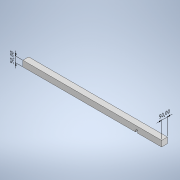
# Autodesk Inventor part: u_lange_Stange
Saved by Autodesk Inventor 2020.3 (Build 243373000, 373)
## iProperties
Created: 2020-09-30
Part Number: u_lange_Stange
Material: Generic
Document SubType Name: Modeling
Designer: Mara
Density: 1 g/cm^3
Appearance: Default
Author: Mara
Autodesk Inventor part; units mm, degrees
ref_plane "YZ Plane" through (0, 0, 0) normal (1, 0, 0) x (0, 1, 0)
ref_plane "XZ Plane" through (0, 0, 0) normal (0, 1, 0) x (-1, 0, 0)
ref_plane "XY Plane" through (0, 0, 0) normal (0, 0, 1) x (1, 0, 0)
sketch "Sketch1" plane through (0, 0, 0) normal (0, 0, 1) x (1, 0, 0)
  line L0 (-600, -25) -> (600, -25)
  line L1 (600, -25) -> (600, 25)
  line L2 (600, 25) -> (-600, 25)
  line L3 (-600, 25) -> (-600, -25)
  line L4 (-600, -25) -> (600, 25) construction
  line L5 (600, -25) -> (-600, 25) construction
  point P0 (0, 0)
  dimension "d0" = 1200
  dimension "d1" = 50
  constraints: 12 end point, 2 midpoint, 2 parallel, 1 horizontal, 1 perpendicular
  measures "d0" distance of L2.end L1.end
  measures "d1" distance of L1.end L0.end
extrude "Extrusion1" add sketch "Sketch1" along normal blind 50
sketch "Sketch2" plane through (0, 0, 0) normal (0, 0, -1) x (-1, 0, 0)
  circle A0 centre (0, 0) radius 9
  circle A1 centre (570, 0) radius 6
  line L0 (600, 25) -> (600, -25) projected
  line L1 (-600, 25) -> (600, 25) projected
  dimension "d13" = 18
  dimension "d20" = 30
  dimension "d21" = 12
  dimension "d22" = 50
  dimension "d23" = 25
  constraints: 2 centre point, 1 coincident
  measures "d13" diameter of A0
  measures "d20" distance from line of L0 A1.centre
  measures "d21" diameter of A1
  measures "d22" distance of L0.start L0.end
  measures "d23" distance from line of L1 A1.centre
extrude "Extrusion2" add sketch "Sketch2" along normal blind 13
sketch "Sketch5" plane through (0, 0, 0) normal (0, 0, -1) x (-1, 0, 0)
  line L0 (600, -25) -> (-600, -25) projected
  line L1 (-391, -25) -> (-391, -3)
  line L2 (-391, -3) -> (-380, -3)
  line L3 (-380, -3) -> (-380, -25) construction
  line L4 (-380, -3) -> (-374.1051, -25)
  point P0 (0, 0)
  dimension "d30" = 15
  dimension "d31" = 22
  dimension "d32" = 11
  dimension "d33" = 209
  constraints: 8 end point, 3 point on line, 2 perpendicular, 1 vertical
  measures "d30" angle of L3 L4
  measures "d31" distance between parallel lines of L0 L2
  measures "d32" distance of L1.end L2.end
  measures "d33" distance of L0.end L1.start
extrude "Extrusion4" cut sketch "Sketch5" against normal through all
equation "\"d23\" = 0.5 * d22"
body "Solid1"
